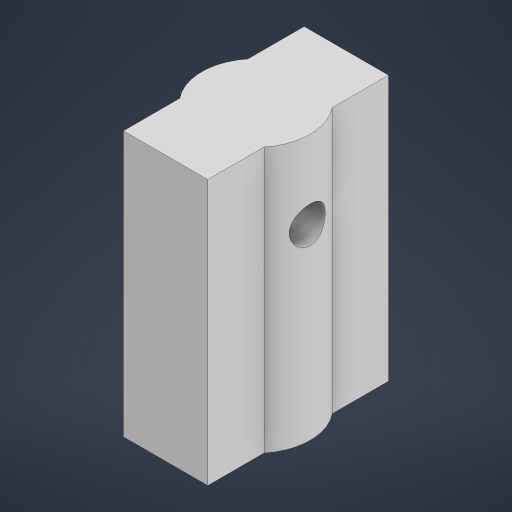
# Autodesk Inventor part: simpleste Anbindung
Saved by Autodesk Inventor 2023.2 (Build 272271000, 271)
## iProperties
Created: 2023-04-05
Part Number: simpleste Anbindung
Material: Generisch
Document SubType Name: Modeling
Designer: tadeus
Density: 1 g/cm^3
Appearance: Vorgabe
Author: tadeus
Autodesk Inventor part; units mm, degrees
ref_plane "YZ Plane" through (0, 0, 0) normal (1, 0, 0) x (0, 1, 0)
ref_plane "XZ Plane" through (0, 0, 0) normal (0, 1, 0) x (-1, 0, 0)
ref_plane "XY Plane" through (0, 0, 0) normal (0, 0, 1) x (1, 0, 0)
sketch "Skizze1" plane through (0, 0, 0) normal (0, 1, 0) x (-1, 0, 0)
  line L0 (3.5, 7.5) -> (-3.5, 7.5)
  line L1 (-3.5, 7.5) -> (-3.5, 2.8284)
  line L2 (-3.5, -7.5) -> (3.5, -7.5)
  line L3 (3.5, -7.5) -> (3.5, -2.8284)
  line L4 (3.5, 7.5) -> (-3.5, -7.5) construction
  line L5 (-3.5, 7.5) -> (3.5, -7.5) construction
  line L6 (-3.5, -2.8284) -> (-3.5, -7.5)
  arc A0 (-3.5, 2.8284) -> (-3.5, -2.8284) centre (0, 0) ccw
  arc A1 (3.5, -2.8284) -> (3.5, 2.8284) centre (0, 0) ccw
  line L7 (3.5, 2.8284) -> (3.5, 7.5)
  line L8 (3.5, -2.8284) -> (3.5, 2.8284) construction
  line L9 (-3.5, -2.8284) -> (-3.5, 2.8284) construction
  arc A2 (-3.5, -2.8284) -> (3.5, -2.8284) centre (0, 0) ccw construction
  arc A3 (3.5, 2.8284) -> (-3.5, 2.8284) centre (0, 0) ccw construction
  dimension "d0" = 7
  dimension "d1" = 15
  dimension "d5" = 4.5
  constraints: 20 end point, 8 point on circle, 6 parallel, 4 centre point, 3 concentric, 2 midpoint, 2 perpendicular, 1 coincident, 1 horizontal, 1 vertical
  measures "d0" distance of L2.end L2.start
  measures "d1" distance of L2.start L0.end
  measures "d5" radius of A2
extrude "Extrusion1" add sketch "Skizze1" along normal blind 22
sketch "Skizze2" plane through (0, 0, 0) normal (1, 0, 0) x (0, 1, 0)
  circle A0 centre (15.5, 0) radius 1.5
  line L0 (0, -7.5) -> (22, -7.5) projected
  line L1 (22, -2.8284) -> (22, 2.8284) projected
  point P0 (0, 0)
  dimension "d8" = 3
  dimension "d9" = 7.5
  dimension "d10" = 6.5
  constraints: 1 centre point
  measures "d8" diameter of A0
  measures "d9" distance from line of L0 A0.centre
  measures "d10" distance from line of L1 A0.centre
extrude "Extrusion2" cut sketch "Skizze2" along normal through all both and the other way through all
